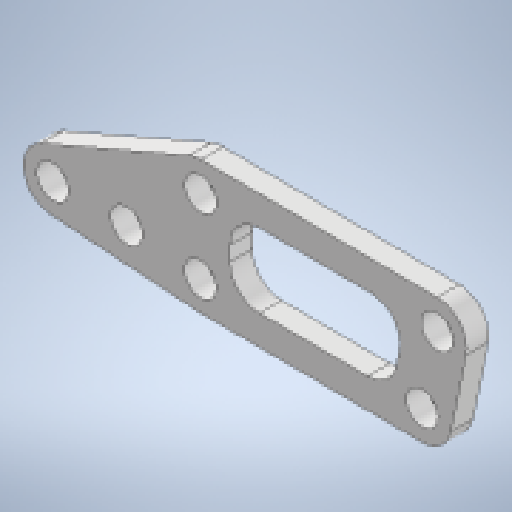
# Autodesk Inventor part: ude_tunagi
Saved by Autodesk Inventor 2025.1 (Build 291241000, 241)
## iProperties
Created: 2024-09-09
Part Number: ude_tunagi
Material: アルミニウム 2014-T4
Document SubType Name: Modeling
Designer: right
Mass: 0.640778 g
Surface Area: 5.15849 cm^2
Volume: 0.228849 cm^3
Density: 2.8 g/cm^3
Appearance: サテン
Author: right
Autodesk Inventor part; units mm, degrees
ref_plane "YZ Plane" through (0, 0, 0) normal (1, 0, 0) x (0, 1, 0)
ref_plane "XZ Plane" through (0, 0, 0) normal (0, 1, 0) x (-1, 0, 0)
ref_plane "XY Plane" through (0, 0, 0) normal (0, 0, 1) x (1, 0, 0)
sketch "スケッチ1" plane through (0, 0, 0) normal (0, 0, 1) x (1, 0, 0)
  circle A0 centre (7.9111, 33.2072) radius 1.1
  circle A1 centre (8.9353, 38.2023) radius 1.1
  circle A2 centre (-7.0645, 38.2798) radius 1.1
  circle A3 centre (-7.0888, 33.2799) radius 1.1
  spline S0 degree 3 poles (-12.8646, 33.9313) (-12.8659, 33.8333) (-12.8476, 33.7285) (-12.7708, 33.5355) (-12.7123, 33.4473) (-12.5725, 33.3024) (-12.4805, 33.2392) (-12.2855, 33.1578) (-12.1826, 33.1393) (-11.9746, 33.1367) (-11.8589, 33.1621) (-11.6558, 33.2543) (-11.5682, 33.3207) (-11.4449, 33.4571) (-11.3945, 33.5329) (-11.3402, 33.6628) (-11.3255, 33.7089) (-11.3046, 33.8062) (-11.2984, 33.8576) (-11.2971, 33.9662) (-11.302, 34.0177) (-11.3205, 34.1156) (-11.334, 34.1619) (-11.3851, 34.2932) (-11.4336, 34.3702) (-11.5535, 34.5096) (-11.6394, 34.5782) (-11.8401, 34.6754) (-11.9552, 34.7036) (-12.1632, 34.7062) (-12.2665, 34.6902) (-12.4635, 34.6136) (-12.557, 34.5528) (-12.7004, 34.4113) (-12.7611, 34.3246) (-12.8426, 34.1336) (-12.8634, 34.0293) (-12.8646, 33.9313) knots 0 0 0 0 0.029408 0.029408 0.058816 0.058816 0.090592 0.090592 0.122368 0.122368 0.162647 0.162647 0.202927 0.202927 0.235498 0.235498 0.251784 0.251784 0.26807 0.26807 0.284355 0.284355 0.300641 0.300641 0.333213 0.333213 0.373492 0.373492 0.413772 0.413772 0.445548 0.445548 0.477323 0.477323 0.506731 0.506731 0.536139 0.536139 0.536139 0.536139
  circle A4 centre (-17.0808, 33.9834) radius 0.7835
  arc A5 (-11.6308, 33.2805) -> (-11.6151, 34.5514) centre (-12.0812, 33.9216) ccw construction
  circle A6 centre (-12.0812, 33.9216) radius 1.1
  circle A7 centre (-17.0808, 33.9834) radius 1.1
  circle A8 centre (8.9353, 38.2023) radius 2
  circle A9 centre (-7.0645, 38.2798) radius 2
  circle A10 centre (-7.0888, 33.2799) radius 2
  circle A11 centre (7.9111, 33.2072) radius 2
  circle A12 centre (-12.0812, 33.9216) radius 2
  circle A13 centre (-17.0808, 33.9834) radius 2
  line L0 (8.945, 40.2023) -> (-7.0548, 40.2798)
  line L1 (9.8703, 32.8055) -> (10.8945, 37.8006)
  line L2 (7.9014, 31.2072) -> (-7.0985, 31.2799)
  line L3 (-7.8529, 40.1179) -> (-17.8692, 35.8215)
  line L4 (-17.2213, 31.9884) -> (-7.2292, 31.2848)
  line L5 (6.9761, 38.604) -> (5.9518, 33.6089)
  line L6 (8.9353, 38.2023) -> (-7.0645, 38.2798)
  line L7 (-5.0888, 33.2702) -> (-5.0645, 38.2701)
  line L8 (-7.0888, 33.2799) -> (7.9111, 33.2072)
  point P0 (0, 0)
  point P1 (-12.8646, 33.9313)
  point P2 (6.9353, 38.212)
  point P3 (6.8957, 38.2122)
  point P4 (5.9111, 33.2169)
extrude "押し出し1" add sketch "スケッチ1" along normal blind 1.5 contours A8 | A8 L5 L6 A9 L0 | L1 A11 L5 L6 A8 | A8 L6 L5 | A9 | A11 | A9 L7 A10 L4 A13 L3 | L2 A10 L8 A11 | A13 | A10 | A12
fillet "フィレット1" radius 2 4 edges at (6.8957, 38.2122, 0.75) (5.9111, 33.2169, 0.75) (-5.0645, 38.2701, 0.75) (-5.0888, 33.2702, 0.75)
